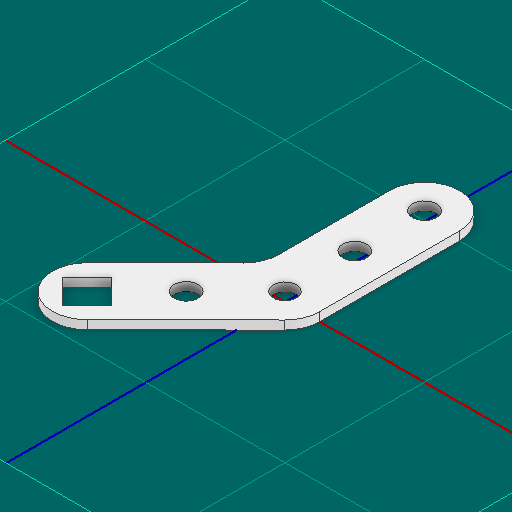
# Autodesk Inventor part: gusset
Saved by Autodesk Inventor 2025 (Build 290162000, 162)
## iProperties
Created: 2024-08-18
Part Number: gusset
Material: Acetal Resin, White
Document SubType Name: Modeling
Designer: averey
Density: 1.425 g/cm^3
Appearance: Smooth - White
d0: 0.500 in
d5: 0.500 in
d6: 0.250 in
d9: 0.248 in
d10: 45.00 deg
d11: 0.248 in
Author: averey
Autodesk Inventor part; units mm, degrees
ref_plane "YZ Plane" through (0, 0, 0) normal (1, 0, 0) x (0, 1, 0)
ref_plane "XZ Plane" through (0, 0, 0) normal (0, 1, 0) x (-1, 0, 0)
ref_plane "XY Plane" through (0, 0, 0) normal (0, 0, 1) x (1, 0, 0)
sketch "main" plane through (0, 0, 0) normal (0, 0, 1) x (1, 0, 0)
  arc A0 (11.6558, 28.6956) -> (2.6985, 37.6987) centre (7.1771, 33.1971) ccw
  circle A1 centre (-10.8061, -10.1403) radius 2.1844
  arc A2 (-17.1561, -10.1402) -> (-4.4561, -10.1282) centre (-10.8061, -10.1403) ccw
  line L0 (2.6985, 37.6987) -> (-15.2847, 19.807)
  circle A3 centre (-1.8258, 24.24) radius 2.1844
  line L1 (11.6558, 28.6956) -> (-2.5847, 14.5275)
  line L2 (-10.8061, 15.2597) -> (27.2939, 15.2597) construction
  circle A4 centre (-10.8061, 2.5597) radius 2.1844
  line L3 (-4.4561, -10.1282) -> (-4.4561, 10.026)
  arc A5 (-2.5847, 14.5275) -> (-4.4561, 10.026) centre (1.8939, 10.026) ccw
  line L4 (-17.1561, -10.1402) -> (-17.1561, 15.3055)
  circle A6 centre (-10.8061, 15.2597) radius 2.0955
  arc A7 (-15.2847, 19.807) -> (-17.1561, 15.3055) centre (-10.8061, 15.3055) ccw
  line L5 (7.1771, 37.6513) -> (11.6313, 33.1971)
  line L6 (11.6313, 33.1971) -> (7.1771, 28.7429)
  line L7 (7.1771, 28.7429) -> (2.7229, 33.1971)
  line L8 (2.7229, 33.1971) -> (7.1771, 37.6513)
  line L9 (7.1771, 37.6513) -> (7.1771, 28.7429) construction
  line L10 (11.6313, 33.1971) -> (2.7229, 33.1971) construction
  line L11 (7.1771, 37.6513) -> (13.4763, 37.6513) construction
  point P0 (0.9467, 22.1756)
  point P1 (5.5442, 34.8331)
  point P2 (8.7899, 34.8537)
  point P3 (5.5158, 31.5901)
  dimension "d0" = 12.7
  dimension "d5" = 12.7
  dimension "d6" = 6.35
  dimension "d9" = 6.2992
  dimension "d10" = 45
  dimension "d11" = 6.2992
  measures "d0" diameter of A2
  measures "d5" diameter of A0
  measures "d6" radius of A7
  measures "d9" distance of L5.start L5.end
  measures "d10" angle of L5 L11
  measures "d11" distance of L5.end L6.end
sketch "Sketch1" plane through (0, 0, 0) normal (0, 1, 0) x (-1, 0, 0)
  arc A0 (22.4619, 13.4358) -> (13.5045, 22.439) centre (17.9832, 17.9374) ccw
  circle A1 centre (0, -25.4) radius 2.1844
  arc A2 (-6.35, -25.4) -> (6.35, -25.3879) centre (0, -25.4) ccw
  line L0 (13.5045, 22.439) -> (-4.4786, 4.5473)
  circle A3 centre (8.9803, 8.9803) radius 2.1844
  line L1 (22.4619, 13.4358) -> (8.2213, -0.7322)
  line L2 (0, 0) -> (38.1, 0) construction
  circle A4 centre (0, -12.7) radius 2.1844
  line L3 (6.35, -25.3879) -> (6.35, -5.2338)
  arc A5 (8.2213, -0.7322) -> (6.35, -5.2338) centre (12.7, -5.2338) ccw
  line L4 (-6.35, -25.4) -> (-6.35, 0.0457)
  circle A6 centre (0, 0) radius 2.0955
  arc A7 (-4.4786, 4.5473) -> (-6.35, 0.0457) centre (0, 0.0457) ccw
  line L5 (17.9832, 22.3916) -> (22.4374, 17.9374)
  line L6 (22.4374, 17.9374) -> (17.9832, 13.4832)
  line L7 (17.9832, 13.4832) -> (13.529, 17.9374)
  line L8 (13.529, 17.9374) -> (17.9832, 22.3916)
  line L9 (17.9832, 22.3916) -> (17.9832, 13.4832) construction
  line L10 (22.4374, 17.9374) -> (13.529, 17.9374) construction
  line L11 (17.9832, 22.3916) -> (24.2824, 22.3916) construction
  constraints: 1 other
extrude "Extrusion1" add sketch "Sketch1" along normal blind 1.5875
body "Solid1"
